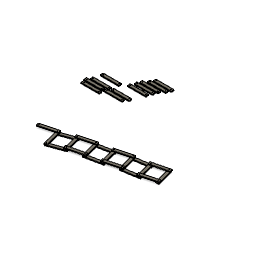
Background Circle Design v1 (Autodesk Fusion 360 design; units mm, degrees)
Autodesk Fusion 360 part; units mm, degrees
sketch "Sketch1" plane through (0, 0, 0) normal (0, 1, 0) x (1, 0, 0)
  line L0 (-31.064, 16.238) -> (68.936, 16.238)
  line L1 (68.936, 16.238) -> (68.936, 1.238)
  line L2 (68.936, 1.238) -> (-31.064, 1.238)
  line L3 (-31.064, 1.238) -> (-31.064, 16.238)
  circle A0 centre (60.936, 8.738) radius 2
  circle A1 centre (-23.064, 8.738) radius 2
  dimension "d3" = 100
  dimension "d4" = 15
  dimension "d7" = 4
  dimension "d8" = 4
  dimension "d9" = 7.5
  dimension "d10" = 7.5
  dimension "d11" = 8
  dimension "d12" = 8
  constraint horizontal L0
  constraint vertical L1
  constraint horizontal L2
  constraint vertical L3
  measures "d3" distance of L0.start L0.end
  measures "d4" distance of L0.start L2.end
  measures "d7" diameter of A1
  measures "d8" diameter of A0
  measures "d9" distance of L0 A1.centre
  measures "d10" distance of L0 A0.centre
  measures "d11" distance of L1 A0.centre
  measures "d12" distance of L3 A1.centre
extrude "Extrude1" add sketch "Sketch1" along normal blind 5 makes body 1
copy_body "CopyPasteBodies1" bodies 1 makes body 2
move_body "Move1" bodies 2 to x (1, 0, 0) y (0, 1, 0) z (0, 0, 1) at (13.6136, 0, -29.6852)
copy_body "Body->Comp1" bodies 1 removing the originals makes body 3 in component "Component"
copy_body "Body->Comp2" bodies 2 removing the originals makes body 4 in component "Component'"
copy_body "CopyPasteBodies2" bodies 4 body 4 seen with x (0.5, 0, -0.866025) y (0, 1, 0) z (0.866025, 0, 0.5) at (14.9367, 5, 2.2893) makes body 5
move_body "Move2" bodies 5 to x (0.5, 0, 0.866025) y (0, 1, 0) z (-0.866025, 0, 0.5) at (66.3864, 0, -80.4996)
copy_body "CopyPasteBodies3" bodies 5 makes body 6
move_body "Move3" bodies 6 to x (1, 0, 0) y (0, 1, 0) z (0, 0, 1) at (-1.3507, 0, 22.061)
copy_body "Body->Comp3" bodies 5 removing the originals makes body 7 in component "Component''"
copy_body "Body->Comp4" bodies 6 removing the originals makes body 8 in component "Component'''"
copy_body "CopyPasteBodies4" bodies 5
copy_body "CopyPasteBodies5" bodies 7 makes body 9
move_body "Move4" bodies 9 to x (1, 0, 0) y (0, 1, 0) z (0, 0, 1) at (-19.3966, 0, -80.4808)
copy_body "CopyPasteBodies6" bodies 7 makes body 10
move_body "Move5" bodies 10 to x (1, 0, 0) y (0, 1, 0) z (0, 0, 1) at (-14.864, 0, -39.3614)
copy_body "Body->Comp5" bodies 9 removing the originals makes body 11 in component "Component''''"
copy_body "CopyPasteBodies7" bodies 10 makes body 12
move_body "Move6" bodies 12 to x (1, 0, 0) y (0, 1, 0) z (0, 0, 1) at (-41.6037, 0, 20.6825)
copy_body "CopyPasteBodies8" bodies 10 makes body 13
move_body "Move7" bodies 13 to x (1, 0, 0) y (0, 1, 0) z (0, 0, 1) at (15.8079, 0, -25.9635)
copy_body "CopyPasteBodies9" bodies 10 makes body 14
move_body "Move8" bodies 14 to x (1, 0, 0) y (0, 1, 0) z (0, 0, 1) at (55.8776, 0, -49.8681)
copy_body "Body->Comp6" bodies 10 removing the originals makes body 15 in component "Component'''''"
copy_body "Body->Comp7" bodies 12 removing the originals makes body 16 in component "Component''''''"
move_body "Move1'" bodies 7 to x (1, 0, 0) y (0, 1, 0) z (0, 0, 1) at (27.2455, 0, 14.0572) in component "Component''"
copy_body "CopyPasteBodies10" bodies 13 makes body 17
move_body "Move9" bodies 17 to x (1, 0, 0) y (0, 1, 0) z (0, 0, 1) at (1.3905, 0, -53.9168)
copy_body "CopyPasteBodies11" bodies 13 makes body 18
move_body "Move10" bodies 18 to x (1, 0, 0) y (0, 1, 0) z (0, 0, 1) at (187.9701, 0, 21.1145)
copy_body "CopyPasteBodies12" bodies 13 makes body 19
move_body "Move11" bodies 19 to x (1, 0, 0) y (0, 1, 0) z (0, 0, 1) at (196.2099, 0, -1.03)
copy_body "CopyPasteBodies13" bodies 13 makes body 20
move_body "Move12" bodies 20 to x (1, 0, 0) y (0, 1, 0) z (0, 0, 1) at (215.2644, 0, -23.6894)
copy_body "CopyPasteBodies14" bodies 13 makes body 21
move_body "Move13" bodies 21 to x (1, 0, 0) y (0, 1, 0) z (0, 0, 1) at (225.5641, 0, -44.2889)
copy_body "CopyPasteBodies15" bodies 13 makes body 22
move_body "Move14" bodies 22 to x (1, 0, 0) y (0, 1, 0) z (0, 0, 1) at (194.665, 0, 41.7139)
copy_body "CopyPasteBodies16" bodies 13 makes body 23
move_body "Move15" bodies 23 to x (1, 0, 0) y (0, 1, 0) z (0, 0, 1) at (204.4497, 0, 60.7684)
copy_body "CopyPasteBodies17" bodies 13 makes body 24
move_body "Move16" bodies 24 to x (1, 0, 0) y (0, 1, 0) z (0, 0, 1) at (212.1745, 0, 80.3379)
copy_body "Body->Comp8" bodies 13 removing the originals makes body 25 in component "Component'''''''"
copy_body "Body->Comp9" bodies 14 removing the originals makes body 26 in component "Component''''''''"
copy_body "Body->Comp10" bodies 17 removing the originals makes body 27 in component "Component'''''''''"
move_body "Move17" bodies 20 24 22 18 21 23 19 to x (1, 0, 0) y (0, 1, 0) z (0, 0, 1) at (-415.7649, 0, -118.8663)
copy_body "CopyPasteBodies18" bodies 22 20 23 21 18 19 24 makes body 28 makes body 29 makes body 30 makes body 31 makes body 32 makes body 33 makes body 34
move_body "Move18" bodies 28 29 30 31 32 33 34 to x (1, 0, 0) y (0, 1, 0) z (0, 0, 1) at (117.3586, 0, 0.0353)
copy_body "CopyPasteBodies19" bodies 22 20 23 21 18 19 24 makes body 35 makes body 36 makes body 37 makes body 38 makes body 39 makes body 40 makes body 41
move_body "Move19" bodies 35 36 37 38 39 40 41 to x (1, 0, 0) y (0, 1, 0) z (0, 0, 1) at (233.6132, 0, -0.0821)
copy_body "Body->Comp11" bodies 18 removing the originals makes body 42 in component "Component''''''''''"
copy_body "Body->Comp12" bodies 19 removing the originals makes body 43 in component "Component'''''''''''"
copy_body "Body->Comp13" bodies 20 removing the originals makes body 44 in component "Component''''''''''''"
move_body "Move20" bodies 33 29 to x (1, 0, 0) y (0, 1, 0) z (0, 0, 1) at (-112.913, 0, 0.6642)
move_body "Move21" bodies 31 to x (1, 0, 0) y (0, 1, 0) z (0, 0, 1) at (-158.0783, 0, 65.7552)
move_body "Move22" bodies 28 32 to x (1, 0, 0) y (0, 1, 0) z (0, 0, 1) at (-204.5719, 0, -65.091)
move_body "Move23" bodies 34 37 to x (1, 0, 0) y (0, 1, 0) z (0, 0, 1) at (-346.7094, 0, -59.1133)
move_body "Move24" bodies 34 to x (1, 0, 0) y (0, 1, 0) z (0, 0, 1) at (94.3156, 0, 1.9926)
move_body "Move25" bodies 35 30 to x (1, 0, 0) y (0, 1, 0) z (0, 0, 1) at (-344.7169, 0, 3.9852)
move_body "Move26" bodies 30 to x (1, 0, 0) y (0, 1, 0) z (0, 0, 1) at (118.2266, 0, 5.9777)
move_body "Move27" bodies 33 24 28 21 37 30 32 31 23 22 34 29 35 to x (1, 0, 0) y (0, 1, 0) z (0, 0, 1) at (-119.555, 0, -53.7997)
move_body "Move28" bodies 38 36 39 41 40 to x (1, 0, 0) y (0, 1, 0) z (0, 0, 1) at (-340.0675, 0, -201.2509)
move_body "Move29" bodies 38 40 39 36 to x (1, 0, 0) y (0, 1, 0) z (0, 0, 1) at (33.8739, 0, 32.5455)
copy_body "Body->Comp14" bodies 21 removing the originals makes body 45 in component "Component'''''''''''''"
copy_body "Body->Comp15" bodies 22 removing the originals makes body 46 in component "Component''''''''''''''"
copy_body "Body->Comp16" bodies 23 removing the originals makes body 47 in component "Component'''''''''''''''"
copy_body "Body->Comp17" bodies 24 removing the originals makes body 48 in component "Component''''''''''''''''"
copy_body "Body->Comp18" bodies 28 removing the originals makes body 49 in component "Component'''''''''''''''''"
copy_body "Body->Comp19" bodies 29 removing the originals makes body 50 in component "Component''''''''''''''''''"
copy_body "Body->Comp20" bodies 30 removing the originals makes body 51 in component "Component'''''''''''''''''''"
copy_body "Body->Comp21" bodies 31 removing the originals makes body 52 in component "Component''''''''''''''''''''"
component "Component" placed x (0.941672, 0, -0.336533) y (0, 1, 0) z (0.336533, 0, 0.941672) at (-200.0169, 0, 9.0989)
component "Component'" placed x (0.248917, 0, 0.968525) y (0, 1, 0) z (-0.968525, 0, 0.248917) at (-259.5377, 5, 27.3495)
component "Component''" placed x (0.941672, 0, -0.336533) y (0, 1, 0) z (0.336533, 0, 0.941672) at (-257.652, -5, 205.6545)
component "Component'''" placed x (0.248917, 0, 0.968525) y (0, 1, 0) z (-0.968525, 0, 0.248917) at (-240.9535, 0, -58.1794)
component "Component''''" placed x (-0.968264, 0, 0.249928) y (0, 1, 0) z (-0.249928, 0, -0.968264) at (-68.8995, 5, -230.8256)
component "Component'''''" placed x (-0.968264, 0, 0.249928) y (0, 1, 0) z (-0.249928, 0, -0.968264) at (-33.3249, 5, -110.7879)
component "Component''''''" placed x (-0.248917, 0, -0.968525) y (0, 1, 0) z (0.968525, 0, -0.248917) at (77.7831, 0, 15.7456)
component "Component'''''''" placed x (0.979875, 0, -0.19961) y (0, 1, 0) z (0.19961, 0, 0.979875) at (-92.3648, -5, 138.7609)
component "Component''''''''" placed x (-0.248917, 0, -0.968525) y (0, 1, 0) z (0.968525, 0, -0.248917) at (252.6873, 0, 75.8302)
component "Component'''''''''" placed x (-0.979875, 0, 0.19961) y (0, 1, 0) z (-0.19961, 0, -0.979875) at (57.7003, -5, -208.5421)
component "Component''''''''''" placed x (0.966487, 0, -0.256714) y (0, 1, 0) z (0.256714, 0, 0.966487) at (245.7654, 5, 159.3317)
component "Component'''''''''''" placed x (-0.966487, 0, 0.256714) y (0, 1, 0) z (-0.256714, 0, -0.966487) at (-105.2567, 5, -237.8524)
component "Component''''''''''''" placed x (-0.248917, 0, -0.968525) y (0, 1, 0) z (0.968525, 0, -0.248917) at (388.9067, 0, -208.2663)
component "Component'''''''''''''" placed x (-0.987398, 0, 0.158259) y (0, 1, 0) z (-0.158259, 0, -0.987398) at (-122.3566, -5, -435.5055)
component "Component''''''''''''''" placed x (0.968525, 0, -0.248917) y (0, 1, 0) z (0.248917, 0, 0.968525) at (546.6188, 5, 211.7204)
component "Component'''''''''''''''" placed x (0.248917, 0, 0.968525) y (0, 1, 0) z (-0.968525, 0, 0.248917) at (-24.4062, 0, 237.0404)
component "Component''''''''''''''''" placed x (0.987398, 0, -0.158259) y (0, 1, 0) z (0.158259, 0, 0.987398) at (418.2103, -5, 220.4694)
component "Component'''''''''''''''''" placed x (0.968525, 0, -0.248917) y (0, 1, 0) z (0.248917, 0, 0.968525) at (138.1449, 5, 293.4603)
component "Component''''''''''''''''''" placed x (0.248917, 0, 0.968525) y (0, 1, 0) z (-0.968525, 0, 0.248917) at (-27.9707, 0, 222.2003)
component "Component'''''''''''''''''''" placed x (0.968525, 0, -0.248917) y (0, 1, 0) z (0.248917, 0, 0.968525) at (614.698, 5, 77.4969)
component "Component''''''''''''''''''''" placed x (1, 0, 0) y (0, 1, 0) z (0, 0, 1) at (0, 0, 0)
equation "Length = 100 mm"
equation "Width = 15 mm"
equation "d3 = Length"
equation "d4 = Width"
equation "thickness = 5 mm"
equation "bolt = 4 mm"
equation "d7 = bolt"
equation "d8 = bolt"
equation "d13 = thickness"
